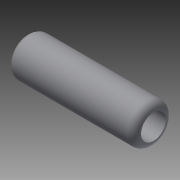
# Autodesk Inventor part: RubberHandleSleeveDE
Saved by Autodesk Inventor 2015 (Build 190159000, 159)
## iProperties
Created: 2017-12-04
Part Number: RubberHandleSleeveDE
Material: Generic
Document SubType Name: Modeling
Designer: Administrator
Density: 1 g/cm^3
Appearance: Default
Author: Administrator
Autodesk Inventor part; units mm, degrees
ref_plane "YZ Plane" through (0, 0, 0) normal (1, 0, 0) x (0, 1, 0)
ref_plane "XZ Plane" through (0, 0, 0) normal (0, 1, 0) x (-1, 0, 0)
ref_plane "XY Plane" through (0, 0, 0) normal (0, 0, 1) x (1, 0, 0)
sketch "Sketch1" plane through (0, 0, 0) normal (0, 0, 1) x (1, 0, 0)
  line L0 (0, 0) -> (0, 15.0812)
  line L1 (0, 15.0812) -> (3.9624, 15.0812)
  line L2 (3.9624, 15.0812) -> (3.9624, 6.35)
  line L3 (3.9624, 6.35) -> (113.5126, 6.35)
  line L4 (113.5126, 6.35) -> (113.5126, 0)
  line L5 (113.5126, 0) -> (0, 0)
  line L6 (0, 17.4625) -> (113.5126, 17.4625)
  dimension "d0" = 15.0813
  dimension "d1" = 8.7312
  dimension "d2" = 6.35
  dimension "d3" = 113.5126
  dimension "d4" = 3.9624
  dimension "d5" = 113.5126
  dimension "d6" = 2.3813
  constraints: 14 end point, 4 perpendicular, 1 horizontal
  measures "d0" distance of L0.start L0.end
  measures "d1" distance of L1.end L2.end
  measures "d2" distance of L3.end L4.end
  measures "d3" distance of L4.end L0.start
  measures "d4" distance of L0.end L1.end
  measures "d5" distance of L6.start L6.end
  measures "d6" distance between parallel lines of L1 L6
revolve "Revolution1" add sketch "Sketch1" angle 360 about axis through (0, 17.4625, 0) along (1, 0, 0)
fillet "Fillet1" radius 6.35 1 edges at (0, 34.925, 0)
fillet "Fillet2" radius 6.35 1 edges at (113.5126, 34.925, 0)
body "Solid1"
